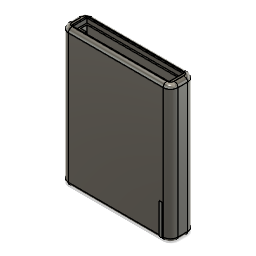
Wemos D1 mini pro Box (Autodesk Fusion 360 design; units mm, degrees)
Autodesk Fusion 360 part; units mm, degrees
sketch "Esquisse1" plane through (0, 0, 0) normal (0, 1, 0) x (1, 0, 0)
  line L0 (-13.2, 2.1) -> (13.2, 2.1)
  line L1 (13.2, 2.1) -> (13.2, -2.1)
  line L2 (13.2, -2.1) -> (-13.2, -2.1)
  line L3 (-13.2, -2.1) -> (-13.2, 2.1)
  line L4 (13.2, 2.1) -> (-13.2, -2.1) construction
  line L5 (-14.8, -3.3) -> (14.8, -3.3)
  line L6 (14.8, -3.3) -> (14.8, 3.3)
  line L7 (14.8, 3.3) -> (-14.8, 3.3)
  line L8 (-14.8, 3.3) -> (-14.8, -3.3)
  line L9 (-4, 1.5) -> (4, 1.5)
  line L10 (4, 1.5) -> (4, -1.5)
  line L11 (4, -1.5) -> (-4, -1.5)
  line L12 (-4, -1.5) -> (-4, 1.5)
  line L13 (0, -1.5) -> (0, 0) construction
  line L14 (-13.2, -0.9) -> (-11.6, -0.9)
  line L15 (11.6, -0.9) -> (13.2, -0.9)
  line L16 (-11.6, -0.9) -> (-11.6, 0.9)
  line L17 (-11.6, 0.9) -> (-13.2, 0.9)
  line L18 (11.6, -0.9) -> (11.6, 0.9)
  line L19 (11.6, 0.9) -> (13.2, 0.9)
  dimension "d1" = 26.4
  dimension "d2" = 4.2
  dimension "d3" = 1.2
  dimension "d4" = 1.2
  dimension "d5" = 1.6
  dimension "d6" = 1.6
  dimension "d7" = 0.6
  dimension "d8" = 8
  dimension "d9" = 3
  dimension "d14" = 1.2
  dimension "d16" = 1.2
  dimension "d41" = 1.6
  constraint horizontal L0
  constraint vertical L1
  constraint horizontal L2
  constraint vertical L3
  constraint midpoint L13.end L4
  constraint horizontal L5
  constraint vertical L6
  constraint horizontal L7
  constraint vertical L8
  constraint horizontal L9
  constraint vertical L10
  constraint horizontal L11
  constraint vertical L12
  constraint midpoint L11 L13.start
  constraint coincident L13.end origin
  constraint vertical L13
  constraint coincident L3 L14.start
  constraint perpendicular L3 L14
  constraint coincident L1 L15.end
  constraint perpendicular L1 L15
  constraint collinear L14 L15
  constraint equal L14 L15
  constraint perpendicular L14 L16
  constraint coincident L3 L17.end
  constraint perpendicular L3 L17
  constraint perpendicular L15 L18
  constraint coincident L1 L19.end
  constraint perpendicular L1 L19
  constraint collinear L17 L19
  measures "d1" distance of L0.start L0.end
  measures "d2" distance of L0 L2
  measures "d3" distance of L0 L7
  measures "d4" distance of L2 L5
  measures "d5" distance of L1 L6
  measures "d6" distance of L3 L8
  measures "d7" distance of L2 L11
  measures "d8" distance of L9.start L9.end
  measures "d9" distance of L9 L11
  measures "d14" distance of L2 L15
  measures "d16" distance of L0 L19
  measures "d41" distance of L1 L18
extrude "Extrusion1" add sketch "Esquisse1" against normal blind 1 contours L0 L1 L2 L3 L14 L15 L16 L17 L18 L19 | L3 L14 L16 L17 | L1 L15 L18 L19 | L5 L6 L7 L8
extrude "Extrusion2" add sketch "Esquisse1" along normal blind 36 contours L5 L6 L7 L8
extrude "Extrusion3" add sketch "Esquisse1" along normal blind 34 contours L3 L14 L16 L17
extrude "Extrusion5" add sketch "Esquisse1" along normal blind 13 from surface at 15 contours L1 L15 L18 L19
sketch "Esquisse6" plane through (0, 0, -3.3) normal (0, 0, -1) x (-1, 0, 0)
  line L0 (-14.8, 36) -> (-14.8, -1)
  line L1 (-14.8, -1) -> (14.8, -1)
  line L2 (14.8, -1) -> (14.8, 36)
  line L3 (14.8, 36) -> (-14.8, 36)
  circle A0 centre (7.1, 28.5) radius 1.25
  point P0 (13.2, 34)
  dimension "d61" = 6.1
  dimension "d62" = 5.5
  dimension "d63" = 2.5
  measures "d61" horizontal distance of A0.centre P0
  measures "d62" vertical distance of A0.centre P0
  measures "d63" diameter of A0
extrude "Extrusion10" cut sketch "Esquisse6" against normal blind 2 contours A0
chamfer "Chanfrein10" distance 1 angle 45 1 edges at (-5.9346, 28.952, -3.3)
fillet "Congé1" radius 2 4 edges at (14.8, 17.5, 3.3) (14.8, 17.5, -3.3) (-14.8, 17.5, 3.3) (-14.8, 17.5, -3.3)
fillet "Congé2" radius 1 8 edges at (14.2142, -1, -2.7142) (14.8, -1, 0) (14.2142, -1, 2.7142) (0, -1, 3.3) (-14.2142, -1, 2.7142) (-14.8, -1, 0) (-14.2142, -1, -2.7142) (0, -1, -3.3)
fillet "Congé3" radius 1 8 edges at (-14.2142, 36, -2.7142) (-14.8, 36, 0) (-14.2142, 36, 2.7142) (0, 36, 3.3) (14.2142, 36, 2.7142) (14.8, 36, 0) (14.2142, 36, -2.7142) (0, 36, -3.3)
chamfer "Chanfrein3" distance 1.6 angle 45 1 edges at (13.2, 15, 0)
chamfer "Chanfrein4" distance 0.5 distance2 2 4 edges at (12.4, 28, -0.9) (12.4, 28, 0.9) (-12.4, 34, -0.9) (-12.4, 34, 0.9) measured on face at (12.6667, 28, 0.3) measured on face at (12.6667, 28, 0.3) measured on face at (-12.6667, 34, -0.3) measured on face at (-12.6667, 34, -0.3)
sketch "Esquisse3" plane through (0, 0, -3.3) normal (0, 0, -1) x (-1, 0, 0)
  line L0 (12.8, 35) -> (-12.8, 35)
  line L1 (-12.8, 35) -> (-12.8, 0)
  line L2 (-12.8, 0) -> (12.8, 0)
  line L3 (12.8, 0) -> (12.8, 35)
  line L4 (-12.5, -2) -> (-11.7, -2)
  line L5 (-11.7, -2) -> (-11.7, 8)
  line L6 (-11.7, 8) -> (-12.5, 8)
  line L7 (-12.5, 8) -> (-12.5, -2)
  circle A0 centre (7.1, 28.5) radius 2.25
  dimension "d35" = 10
  dimension "d36" = 12.5
  dimension "d37" = 0.8
  dimension "d38" = 2
  constraint horizontal L4
  constraint vertical L5
  constraint horizontal L6
  constraint vertical L7
  measures "d35" distance of L4.start L6.end
  measures "d36" distance of origin L7
  measures "d37" distance of L5 L7
  measures "d38" distance of origin L4
extrude "Extrusion6" cut sketch "Esquisse3" against normal blind 21 contours L2 L4 L5 L7 | L2 L5 L6 L7
sketch "Esquisse4" plane through (13.2, 0, 0) normal (-1, 0, 0) x (0, 0, 1)
  line L0 (-0.9, 13.4) -> (-0.9, 26)
  line L1 (-0.9, 26) -> (-0.4, 28)
  line L2 (-0.4, 28) -> (0.4, 28)
  line L3 (0.4, 28) -> (0.9, 26)
  line L4 (0.9, 26) -> (0.9, 13.4)
  line L5 (0.9, 13.4) -> (-0.9, 13.4)
  line L6 (-2.1, 0) -> (2.1, 0)
  line L7 (2.1, 0) -> (2.1, 36)
  line L8 (2.1, 36) -> (-2.1, 36)
  line L9 (-2.1, 36) -> (-2.1, 0)
  line L10 (1.5, 0) -> (-1.5, 0)
  line L11 (-1.5, 0) -> (-1.5, 5)
  line L12 (-1.5, 5) -> (1.5, 5)
  line L13 (1.5, 5) -> (1.5, 0)
  line L14 (1.5, 0.4) -> (-1.5, 0.4)
  line L15 (-1.5, 5) -> (-2.1, 5)
  line L16 (1.5, 5) -> (2.1, 5)
  dimension "d42" = 5
  dimension "d43" = 0.6
  dimension "d44" = 0.6
  dimension "d45" = 0.4
  constraint horizontal L10
  constraint vertical L11
  constraint horizontal L12
  constraint vertical L13
  constraint coincident L6 L10.start
  constraint coincident L13 L14.start
  constraint coincident L11 L14.end
  constraint perpendicular L11 L14
  constraint coincident L9 L15.end
  constraint perpendicular L9 L15
  constraint coincident L7 L16.end
  constraint perpendicular L7 L16
  measures "d42" distance of origin L12
  measures "d43" distance of L9 L11
  measures "d44" distance of L7 L13
  measures "d45" distance of L10 L14
extrude "Extrusion7" add sketch "Esquisse4" along normal blind 2 contours L11 L12 L13 L14
chamfer "Chanfrein5" distance 1 angle 45 1 edges at (11.2, 5, 0)
extrude "Extrusion8" add sketch "Esquisse4" along normal blind 0.7 contours L6 L9 L11 L15 | L6 L10 L11 L13 L14 | L6 L7 L13 L16
chamfer "Chanfrein6" distance 0.6 distance2 1.4 1 edges at (12.5, 0.4, 0) measured on face at (11.6333, 0.4, -0.5)
chamfer "Chanfrein7" distance 0.3 angle 45 1 edges at (11.9, 0.4, 0)
chamfer "Chanfrein8" distance 0.8 angle 45 2 edges at (12.5, 2, 1.5) (12.5, 2, -1.5)
sketch "Esquisse7" plane through (0, 36, 0) normal (0, 1, 0) x (-1, 0, 0)
  line L0 (-13.2, 2.1) -> (13.2, 2.1)
  line L1 (13.2, 2.1) -> (13.2, -2.1)
  line L2 (13.2, -2.1) -> (-13.2, -2.1)
  line L3 (-13.2, -2.1) -> (-13.2, 2.1)
  arc A0 (12.8, -2.3) -> (13.8, -1.3) centre (12.8, -1.3) ccw
  line L4 (13.8, -1.3) -> (13.8, 1.3)
  arc A1 (13.8, 1.3) -> (12.8, 2.3) centre (12.8, 1.3) ccw
  line L5 (12.8, 2.3) -> (-12.8, 2.3)
  arc A2 (-12.8, 2.3) -> (-13.8, 1.3) centre (-12.8, 1.3) ccw
  line L6 (-13.8, 1.3) -> (-13.8, -1.3)
  arc A3 (-13.8, -1.3) -> (-12.8, -2.3) centre (-12.8, -1.3) ccw
  line L7 (-12.8, -2.3) -> (12.8, -2.3)
extrude "Extrusion11" cut sketch "Esquisse7" against normal blind 1.6 draft 15 from surface at -0.4 contours L0 L1 L2 L3
chamfer "Chanfrein11" distance 0.4 angle 45 1 edges at (11.7, 0, 0)
sketch "Esquisse8" plane through (0, 0, 0) normal (0, 1, 0) x (-1, 0, 0)
  line L0 (-11.3, 2.1) -> (-11.3, -2.1)
  line L1 (-11.3, -2.1) -> (13.2, -2.1)
  line L2 (13.2, -2.1) -> (13.2, -0.9)
  line L3 (13.2, -0.9) -> (11.6, -0.9)
  line L4 (11.6, -0.9) -> (11.6, 0.9)
  line L5 (11.6, 0.9) -> (13.2, 0.9)
  line L6 (13.2, 0.9) -> (13.2, 2.1)
  line L7 (13.2, 2.1) -> (-11.3, 2.1)
  line L8 (-4, 1.5) -> (4, 1.5)
  line L9 (4, 1.5) -> (4, -1.5)
  line L10 (4, -1.5) -> (-4, -1.5)
  line L11 (-4, -1.5) -> (-4, 1.5)
  line L12 (4, 0.1) -> (6, 0.1)
  line L13 (6, 0.1) -> (6, -2.1)
  line L14 (-4, 0.1) -> (-6, 0.1)
  line L15 (-6, 0.1) -> (-6, -2.1)
  dimension "d73" = 6
  dimension "d75" = 0.1
  constraint coincident L9 L12.start
  constraint perpendicular L9 L12
  constraint coincident L1 L13.end
  constraint perpendicular L1 L13
  constraint coincident L11 L14.start
  constraint perpendicular L11 L14
  constraint coincident L1 L15.end
  constraint perpendicular L1 L15
  constraint collinear L12 L14
  constraint equal L12 L14
  measures "d73" distance of origin L15
  measures "d75" distance of origin L14
extrude "Extrusion13" add sketch "Esquisse8" along normal blind 3 contours L1 L9 L10 L11 L12 L13 L14 L15
chamfer "Chanfrein12" distance 0.6 distance2 1.5 7 edges at (-5, 3, 0.1) (-4, 3, -0.7) (0, 3, -1.5) (-6, 3, -1) (6, 3, -1) (4, 3, -0.7) (5, 3, 0.1) measured on face at (-5.3333, 3, -1.1667) measured on face at (-5.3333, 3, -1.1667) measured on face at (-5.3333, 3, -1.1667) measured on face at (-5.3333, 3, -1.1667) measured on face at (-5.3333, 3, -1.1667) measured on face at (-5.3333, 3, -1.1667) measured on face at (-5.3333, 3, -1.1667)
chamfer "Chanfrein13" distance 1 angle 45 2 edges at (-6, 0.75, 0.1) (6, 0.75, 0.1)
chamfer "Chanfrein14" distance 0.4 angle 45 4 edges at (4, -1, 0) (0, -1, 1.5) (0, -1, -1.5) (-4, -1, 0)
sketch "Esquisse9" plane through (0, 0, 2.1) normal (0, 0, -1) x (-1, 0, 0)
  line L0 (13.2, 34) -> (-13.2, 34)
  line L1 (-13.2, 34) -> (-13.2, 5)
  line L2 (-13.2, 5) -> (-12.3, 5)
  line L3 (-12.3, 5) -> (-12.3, 8)
  line L4 (-12.3, 8) -> (-11.7, 8)
  line L5 (-11.7, 8) -> (-11.7, -0.4)
  line L6 (-11.7, -0.4) -> (-11.3, 0)
  line L7 (-11.3, 0) -> (13.2, 0)
  line L8 (13.2, 0) -> (13.2, 34)
  line L9 (-1.5, 19) -> (1.5, 19)
  line L10 (1.5, 19) -> (1.5, 15)
  line L11 (1.5, 15) -> (-1.5, 15)
  line L12 (-1.5, 15) -> (-1.5, 19)
  line L13 (0, 0) -> (0, 15) construction
  dimension "d82" = 15
  dimension "d83" = 3
  dimension "d84" = 4
  constraint horizontal L9
  constraint vertical L10
  constraint horizontal L11
  constraint vertical L12
  constraint coincident L13.start origin
  constraint midpoint L11 L13.end
  constraint vertical L13
  measures "d82" distance of L13.start L13.end
  measures "d83" distance of L9.start L9.end
  measures "d84" distance of L9 L11
extrude "Extrusion14" add sketch "Esquisse9" along normal blind 0.3 contours L9 L10 L11 L12
chamfer "Chanfrein15" distance 1 distance2 0.3 1 faces at (0.5, 17.6667, 1.8)
equation "d30 = 28 mm - 15 mm"
